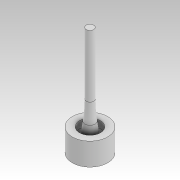
# Autodesk Inventor part: FlowSimulator
Saved by Autodesk Inventor 2020 (Build 240168000, 168)
## iProperties
Created: 2021-09-15
Part Number: FlowSimulator
Material: Generic
Document SubType Name: Modeling
Designer: DDeGo
Density: 1 g/cm^3
Appearance: Default
Author: DDeGo
Autodesk Inventor part; units mm, degrees
ref_plane "YZ Plane" through (0, 0, 0) normal (1, 0, 0) x (0, 1, 0)
ref_plane "XZ Plane" through (0, 0, 0) normal (0, 1, 0) x (-1, 0, 0)
ref_plane "XY Plane" through (0, 0, 0) normal (0, 0, 1) x (1, 0, 0)
sketch "Sketch1" plane through (0, 0, 0) normal (0, 0, 1) x (1, 0, 0)
  line L0 (1.5, -5) -> (-1.5, -5) construction
  line L1 (-1.5, -3) -> (-1.0682, 0.2078)
  line L2 (-0.8, 4.2102) -> (-0.8, 17.2)
  line L3 (0, 0) -> (0, 3.0594) construction
  arc A0 (-1.0682, 0.2078) -> (-0.8, 4.2102) centre (-30.8, 4.2102) ccw
  line L4 (-1.5, -3) -> (0, -3) construction
  line L5 (0, -3) -> (0, 0)
  line L6 (-0.8, 17.2) -> (0, 17.2)
  line L7 (0, 17.2) -> (0, 0)
  line L8 (-1.5, -3) -> (-2.2, -2.3)
  line L9 (-2.2, -2.3) -> (-2.2, -0.8)
  line L10 (-2.2, -0.8) -> (-3.7, -0.8)
  line L11 (-3.7, -0.8) -> (-3.7, -5.5)
  line L12 (-3.7, -5.5) -> (-2.5, -5.5)
  line L13 (-2.5, -5.5) -> (-2.5, -4)
  line L14 (-2.5, -4) -> (0, -4)
  line L15 (0, -4) -> (0, -3)
  point P0 (-0.8, 2.2)
  dimension "d0" = 0.8
  dimension "d2" = 15
  dimension "d4" = 30
  dimension "d6" = 1.5
  dimension "d9" = 5.2
  dimension "d10" = 3
  dimension "d11" = 135
  dimension "d12" = 1.5
  dimension "d13" = 1.5
  dimension "d14" = 1
  dimension "d15" = 1.5
  dimension "d16" = 2.5
  dimension "d17" = 0.7
  constraints: 32 end point, 7 perpendicular, 3 vertical, 2 horizontal, 2 point on circle, 2 point on line, 2 tangent, 1 centre point, 1 coincident
  measures "d0" distance between parallel lines of L3 L2
  measures "d2" distance of point (-0.8, 2.2) L2.end
  measures "d4" radius of A0
  measures "d6" distance of L1.start L4.end
  measures "d9" distance from line of L4 point (-0.8, 2.2)
  measures "d10" distance of L4.end L3.start
  measures "d11" angle of L4 L8
  measures "d12" distance of L8.end L9.end
  measures "d13" distance of L9.end L10.end
  measures "d14" distance between parallel lines of L4 L14
  measures "d15" distance between parallel lines of L14 L12
  measures "d16" distance between parallel lines of L15 L13
  measures "d17" distance from line of L8.end L4
revolve "Revolution1" add sketch "Sketch1" angle 360 about axis through (0, 0, 0) along (0, 1, 0)
body "Solid1"
